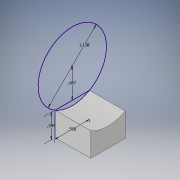
# Autodesk Inventor part: repose rond tournant 1
Saved by Autodesk Inventor 2017 (Build 210142000, 142)
## iProperties
Created: 2018-11-16
Part Number: repose rond tournant 1
Material: Generic
Document SubType Name: Modeling
Designer: Antoine Blaud
Density: 1 g/cm^3
Appearance: Default
Author: Antoine Blaud
Autodesk Inventor part; units mm, degrees
ref_plane "YZ Plane" through (0, 0, 0) normal (1, 0, 0) x (0, 1, 0)
ref_plane "XZ Plane" through (0, 0, 0) normal (0, 1, 0) x (-1, 0, 0)
ref_plane "XY Plane" through (0, 0, 0) normal (0, 0, 1) x (1, 0, 0)
sketch "Sketch1" plane through (0, 0, 0) normal (1, 0, 0) x (0, 1, 0)
  line L0 (0, 0) -> (10, 0)
  line L1 (10, 0) -> (10, -14.4272)
  line L2 (10, -14.4272) -> (0, -14.4272)
  line L3 (0, -14.4272) -> (0, 0)
  circle A0 centre (22.3795, -7.2136) radius 14.3279
  dimension "d3" = 28.6558
  dimension "d0" = 10
  dimension "d1" = 14.4272
  dimension "d4" = 12.3795
  constraints: 8 end point, 2 parallel, 1 horizontal, 1 perpendicular, 3 other
  measures "d0" distance between parallel lines of L1 L3
  measures "d1" distance between parallel lines of L0 L2
  measures "d4" distance from line of point (22.38, -7.214) L1
extrude "Extrusion1" add sketch "Sketch1" along normal blind 15 contours L0 A0 L2 L3 | L1 A0 picked at (9.5878, -8.7004)
extrude "Extrusion2" cut sketch "Sketch1" along normal blind 40 contours A0 L1 | L1 A0
body "Solid1"
